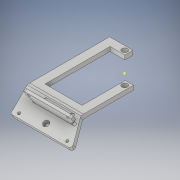
# Autodesk Inventor part: burnisher_cameras_mount
Saved by Autodesk Inventor 2019 (Build 230136000, 136)
## iProperties
Created: 2019-11-07
Part Number: burnisher_cameras_mount
Material: Generic
Document SubType Name: Modeling
Designer: luua
Density: 1 g/cm^3
Appearance: Default
Author: luua
Autodesk Inventor part; units mm, degrees
sketch "Sketch1" plane through (0, 0, 0) normal (0, 1, 0) x (-1, 0, 0)
  circle A0 centre (-17.6777, 17.6777) radius 3.3
  circle A1 centre (-17.6777, -17.6777) radius 3.25 construction
  circle A2 centre (17.6777, -17.6777) radius 3.3
  circle A3 centre (17.6777, 17.6777) radius 3.25 construction
  circle A4 centre (25, 0) radius 3 construction
  circle A5 centre (0, 0) radius 30.5 construction
  circle A6 centre (0, 0) radius 16.75 construction
  line L0 (40, -22.4277) -> (12.9277, -22.4277)
  line L1 (12.9277, -22.4277) -> (12.9277, -12.9277)
  line L2 (12.9277, -12.9277) -> (30, -12.9277)
  line L3 (30, -12.9277) -> (30, 62.5)
  line L4 (30, 62.5) -> (-12.9277, 62.5)
  line L5 (-12.9277, 62.5) -> (-12.9277, 12.3777)
  line L6 (-12.9277, 12.3777) -> (-22.4277, 12.3777)
  line L7 (-22.4277, 12.3777) -> (-22.4277, 71.7952)
  line L8 (40, -22.4277) -> (40, 71.7952)
  line L9 (32.5, 32.5) -> (-32.5, 32.5) construction
  line L10 (-32.5, 32.5) -> (-32.5, -32.5) construction
  line L11 (-32.5, -32.5) -> (32.5, -32.5) construction
  line L12 (32.5, -32.5) -> (32.5, 32.5) construction
  line L13 (32.5, 32.5) -> (-32.5, -32.5) construction
  line L14 (-32.5, 32.5) -> (32.5, -32.5) construction
  line L15 (20, 32.5) -> (20, 57.5) construction
  line L16 (20, 57.5) -> (-5, 57.5) construction
  line L17 (-5, 57.5) -> (-5, 32.5) construction
  line L18 (5, 57.5) -> (5, 32.5) construction
  line L19 (5, 32.5) -> (-5, 32.5) construction
  line L20 (40, 71.7952) -> (-22.4277, 71.7952)
  point P0 (0, 32.5)
  point P1 (12.9277, -17.6777)
  point P2 (-17.6777, 12.3777)
  dimension "d0" = 65
  dimension "d1" = 65
  dimension "d2" = 10
  dimension "d3" = 15
  dimension "d4" = 25
  dimension "d5" = 2
  dimension "d6" = 5
  dimension "d7" = 4.75
  dimension "d8" = 4.75
  dimension "d9" = 4.75
  dimension "d10" = 10
  dimension "d11" = 10
  dimension "d96" = 6.6
  dimension "d97" = 6.6
  constraints: 42 end point, 9 perpendicular, 7 centre point, 6 midpoint, 4 horizontal, 4 point on line, 3 vertical, 2 horizontal alignment, 2 parallel, 1 collinear, 1 vertical alignment, 13 other
  measures "d0" distance of L11.end L10.end
  measures "d1" distance of L10.end L9.end
  measures "d2" distance between parallel lines of L17 L18
  measures "d3" distance between parallel lines of L15 L18
  measures "d4" distance of L16.end L17.end
  measures "d5" distance edge to line of A0 L6
  measures "d6" distance between parallel lines of L4 L16
  measures "d7" distance from line of A0.centre L5
  measures "d8" distance from line of L0 A2.centre
  measures "d9" distance from line of A2.centre L1
  measures "d10" distance between parallel lines of L8 L3
  measures "d11" distance between parallel lines of L15 L3
  measures "d96" diameter of A0
  measures "d97" diameter of A2
extrude "Extrusion1" add sketch "Sketch1" along normal blind 5
ref_plane "Work Plane1" through (22.4277, 5, 71.7952) normal (0, 0.8660254, 0.5) x (1, 0, 0)
sketch "Sketch4" plane through (22.4277, 5, 71.7952) normal (0, 0.8660254, 0.5) x (1, 0, 0)
  line L0 (-62.4277, 0) -> (0, 0) projected
  line L1 (-23, 20) -> (-23, 0) construction
  circle A0 centre (-51, -25.748) radius 1.5
  circle A1 centre (5, -25.748) radius 1.5
  circle A2 centre (-23, -21.748) radius 3.25
  line L2 (-51, -25.748) -> (5, -25.748) construction
  line L3 (-58, -27.748) -> (-58, -25.748)
  line L4 (0, -2.5) -> (-62.4277, -2.5) projected
  line L5 (-62.4277, 81.5994) -> (-62.4277, 0) projected
  line L6 (-62.4277, -2.5) -> (-62.4277, 79.0994) projected
  line L7 (-62.4277, 0) -> (-62.4277, -2.5)
  line L8 (-62.4277, -2.5) -> (-58, -25.748)
  line L9 (0, 48.9571) -> (0, -2.5) projected
  line L10 (0, 0) -> (0, -2.5)
  line L11 (0, -2.5) -> (12, -25.748)
  line L12 (12, -25.748) -> (12, -27.748)
  line L13 (-56, -29.748) -> (10, -29.748)
  arc A3 (-58, -27.748) -> (-56, -29.748) centre (-56, -27.748) ccw
  arc A4 (10, -29.748) -> (12, -27.748) centre (10, -27.748) ccw
  point P0 (-23, -25.748)
  point P1 (-58, -29.748)
  point P2 (12, -29.748)
  dimension "d43" = 3
  dimension "d44" = 6.5
  dimension "d45" = 4
  dimension "d58" = 4
  dimension "d60" = 70
  dimension "d61" = 2
  dimension "d83" = 56
  constraints: 18 end point, 5 centre point, 5 point on line, 4 point on circle, 4 tangent, 4 vertical, 3 horizontal alignment, 2 equal radius, 2 perpendicular, 2 vertical alignment, 1 coincident, 1 horizontal, 1 midpoint, 1 parallel, 1 other
  measures "d43" diameter of A0
  measures "d44" diameter of A2
  measures "d45" distance from line of L2 A2.centre
  measures "d58" distance from line of L13 L2.start
  measures "d60" distance of point (-58, -29.748) point (12, -29.748)
  measures "d61" radius of A3
  measures "d83" distance of A1.centre L2.start
extrude "Extrusion3" add sketch "Sketch4" against normal blind 5
sketch "Sketch5" plane through (22.4277, 5, 71.7952) normal (0, 0.8660254, 0.5) x (1, 0, 0)
  line L0 (-45.5, -8.698) -> (-0.5, -8.698)
  line L1 (-0.5, -8.698) -> (-0.5, -11.698)
  line L2 (-0.5, -11.698) -> (-45.5, -11.698)
  line L3 (-45.5, -11.698) -> (-45.5, -8.698)
  line L4 (-62.4277, 0) -> (0, 0) projected
  line L5 (-62.4277, 0) -> (-62.4277, -2.5) projected
  line L6 (0, -2.5) -> (0, 0) projected
  line L7 (-62.4277, -2.5) -> (-58, -25.748) projected
  line L8 (-58, -25.748) -> (-58, -27.748) projected
  line L9 (-56, -29.748) -> (10, -29.748) projected
  line L10 (12, -27.748) -> (12, -25.748) projected
  line L11 (12, -25.748) -> (0, -2.5) projected
  arc A0 (-58, -27.748) -> (-56, -29.748) centre (-56, -27.748) ccw projected
  arc A1 (10, -29.748) -> (12, -27.748) centre (10, -27.748) ccw projected
  circle A2 centre (-23, -21.748) radius 3.25 projected
  point P0 (-22.4277, 59.6764)
  point P1 (-23, -11.698)
  dimension "d50" = 3
  dimension "d51" = 45
  dimension "d62" = 10.05
  constraints: 8 end point, 2 parallel, 1 horizontal, 1 midpoint, 1 perpendicular, 1 vertical alignment
  measures "d50" distance of L0.end L1.end
  measures "d51" distance of L0.start L0.end
  measures "d62" distance from line of L2 A2.centre
extrude "Extrusion4" add sketch "Sketch5" along normal blind 4 contours L0 L1 L2 L3
sketch "Sketch7" plane through (22.4277, 8.4641, 73.7952) normal (0, 0.8660254, 0.5) x (1, 0, 0)
  line L0 (-0.5, -8.698) -> (-45.5, -8.698) projected
  line L1 (-45.5, -8.698) -> (-45.5, -11.698) projected
  line L2 (-45.5, -11.698) -> (-0.5, -11.698) projected
  line L3 (-0.5, -11.698) -> (-0.5, -8.698) projected
  line L4 (-50.5, -11.698) -> (4.5, -11.698)
  line L5 (4.5, -11.698) -> (4.5, -8.698)
  line L6 (4.5, -8.698) -> (-50.5, -8.698)
  line L7 (-50.5, -8.698) -> (-50.5, -11.698)
  line L8 (-50.5, -11.698) -> (4.5, -8.698) construction
  line L9 (4.5, -11.698) -> (-50.5, -8.698) construction
  point P0 (-23, -10.198)
  dimension "d85" = 55
  constraints: 12 end point, 2 midpoint, 2 parallel, 1 horizontal, 1 perpendicular
  measures "d85" distance of L6.end L5.end
extrude "Extrusion5" add sketch "Sketch7" along normal blind 12
sketch "Sketch6" plane through (-23.0723, -0.849, 81.9259) normal (0, -0.5, 0.8660254) x (1, 0, 0)
  circle A0 centre (0, 12.5) radius 1.6
  circle A1 centre (45, 12.5) radius 1.6
  line L0 (45, 0) -> (0, 0) projected
  line L1 (45, 0) -> (45, 4) projected
  line L2 (0, 0) -> (0, 4) projected
  line L3 (0, 12.5) -> (45, 12.5) construction
  line L4 (45, 4) -> (50, 4) projected
  line L5 (50, 4) -> (50, 16) projected
  line L6 (-5, 16) -> (50, 16) projected
  line L7 (-5, 4) -> (-5, 16) projected
  line L8 (-5, 4) -> (0, 4) projected
  point P0 (22.5, 16)
  point P1 (22.5, 12.5)
  dimension "d67" = 12.5
  dimension "d74" = 3.2
  dimension "d75" = 3.2
  dimension "d84" = 45
  constraints: 2 centre point, 2 end point, 1 horizontal, 1 horizontal alignment, 1 midpoint, 1 vertical alignment
  measures "d67" distance from line of L0 L3.start
  measures "d74" diameter of A0
  measures "d75" diameter of A1
  measures "d84" distance of L3.end L3.start
extrude "Extrusion6" cut sketch "Sketch6" against normal up to next contours A0 | A1
sketch "Sketch8" plane through (-23.0723, -0.849, 81.9259) normal (0, -0.5, 0.8660254) x (1, 0, 0)
  line L0 (-5, 16) -> (50, 16) projected
  line L1 (22.5, 16) -> (22.5, 0) construction
  line L2 (-16.9277, 0) -> (45.5, 0) projected
  line L3 (0, 0) -> (0, 4) projected
  line L4 (0, 4) -> (-5, 4)
  line L5 (-5, 4) -> (-5, 9)
  line L6 (-5, 4) -> (-5, 16) projected
  line L7 (-5, 9) -> (0, 4)
  line L8 (45, 4) -> (50, 4)
  line L9 (50, 4) -> (50, 9)
  line L10 (50, 9) -> (45, 4)
  point P0 (23.0723, -40.2277)
  dimension "d86" = 5
  constraints: 14 end point, 3 symmetric about line, 2 point on line, 1 horizontal, 1 midpoint, 1 vertical
  measures "d86" distance of L4.end L5.end
extrude "Extrusion7" cut sketch "Sketch8" against normal up to surface (3 mm away)
ref_plane "Work Plane2" through (-0.5723, 14.5074, 87.3278) normal (-1, 0, 0) x (0, -0.5, 0.8660254)
sketch "Sketch9" plane through (-0.5723, 14.5074, 87.3278) normal (-1, 0, 0) x (0, -0.5, 0.8660254)
  line L0 (0, -8) -> (-6, -16)
  line L1 (-6, -16) -> (0, -16)
  line L2 (0, -16) -> (0, -8)
  point P0 (-68.3744, -56.2277)
  dimension "d88" = 8
  dimension "d89" = 6
  constraints: 6 end point, 1 horizontal, 1 perpendicular
  measures "d88" distance of L1.end L0.start
  measures "d89" distance of L0.end L1.end
extrude "Extrusion8" add sketch "Sketch9" along normal mid plane 30
ref_plane "Work Plane3" through (-8.5362, 0, 62.5) normal (1, 0, 0) x (0, 0, -1)
sketch "Sketch10" plane through (-8.5362, 0, 62.5) normal (1, 0, 0) x (0, 0, -1)
  line L0 (-29.0936, -12.2041) -> (-8.9602, -0.5801) projected
  line L1 (-15.866, -4.5672) -> (0, 0)
  line L2 (-7.9554, 0) -> (84.9277, 0) projected
  line L3 (50.1223, 0) -> (-7.9554, 0) projected
  line L4 (0, 0) -> (-7.9554, 0)
  line L5 (-7.9554, 0) -> (-15.866, -4.5672)
  point P0 (62.5, 0)
  point P1 (-9.2952, 0)
  constraints: 6 end point, 2 point on line, 1 collinear
extrude "Extrusion9" add sketch "Sketch10" along normal mid plane 42.928
fillet "Fillet3" radius 2 10 edges at (-28.0723, 13.7574, 88.6269) (26.9277, 13.7574, 88.6269) (-28.0723, 7.6952, 85.1269) (26.9277, 7.6952, 85.1269) (21.9277, 3.3651, 82.6269) (-23.0723, 3.3651, 82.6269) (-23.0723, -0.099, 80.6269) (21.9277, -0.099, 80.6269) (-15.5723, 2.151, 76.7298) (14.4277, 2.151, 76.7298)
fillet "Fillet3" radius 5 1 edges at (-8.7862, 5, 71.7952)
equation "\"d8\" = d7"
equation "\"d9\" = d8"
equation "\"d75\" = d74"
body "Solid1"
